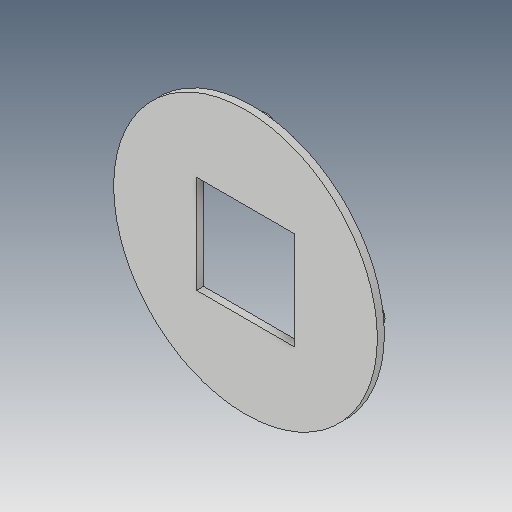
# Autodesk Inventor part: 200_Lambdaplatte_2_conterplate
Saved by Autodesk Inventor 2019 (Build 230136000, 136)
## iProperties
Created: 2019-07-08
Part Number: 200_Lambdaplatte_2_conterplate
Material: Generic
Document SubType Name: Modeling
Designer: diederichbenedict
Density: 1 g/cm^3
Appearance: Default
Author: diederichbenedict
Autodesk Inventor part; units mm, degrees
ref_plane "YZ Plane" through (0, 0, 0) normal (1, 0, 0) x (0, 1, 0)
ref_plane "XZ Plane" through (0, 0, 0) normal (0, 1, 0) x (-1, 0, 0)
ref_plane "XY Plane" through (0, 0, 0) normal (0, 0, 1) x (1, 0, 0)
sketch "Sketch1" plane through (0, 0, 0) normal (0, 0, 1) x (1, 0, 0)
  circle A0 centre (-7.7782, 0) radius 0.9 construction
  circle A1 centre (7.7782, 0) radius 0.9 construction
  circle A2 centre (0, -7.7782) radius 0.9 construction
  circle A3 centre (0, 7.7782) radius 0.9 construction
  arc A4 (0, 10) -> (-2.698, 9.6292) centre (0, 0) ccw construction
  arc A5 (-2.698, 9.6292) -> (-5.1958, 8.5442) centre (0, 0) ccw construction
  arc A6 (-5.1958, 8.5442) -> (-7.3084, 6.8255) centre (0, 0) ccw construction
  arc A7 (-7.3084, 6.8255) -> (-8.8789, 4.6007) centre (0, 0) ccw construction
  arc A8 (-8.8789, 4.6007) -> (-9.7908, 2.0346) centre (0, 0) ccw construction
  arc A9 (-9.7908, 2.0346) -> (-9.9767, -0.6824) centre (0, 0) ccw construction
  arc A10 (-9.9767, -0.6824) -> (-9.4226, -3.3488) centre (0, 0) ccw construction
  arc A11 (-9.4226, -3.3488) -> (-8.1697, -5.7668) centre (0, 0) ccw construction
  arc A12 (-8.1697, -5.7668) -> (-6.3109, -7.7571) centre (0, 0) ccw construction
  arc A13 (-6.3109, -7.7571) -> (-3.984, -9.1721) centre (0, 0) ccw construction
  arc A14 (-3.984, -9.1721) -> (-1.3617, -9.9069) centre (0, 0) ccw construction
  arc A15 (-1.3617, -9.9069) -> (1.3617, -9.9069) centre (0, 0) ccw construction
  arc A16 (1.3617, -9.9069) -> (3.984, -9.1721) centre (0, 0) ccw construction
  arc A17 (3.984, -9.1721) -> (6.3109, -7.7571) centre (0, 0) ccw construction
  arc A18 (6.3109, -7.7571) -> (8.1697, -5.7668) centre (0, 0) ccw construction
  arc A19 (8.1697, -5.7668) -> (9.4226, -3.3488) centre (0, 0) ccw construction
  arc A20 (9.4226, -3.3488) -> (9.9767, -0.6824) centre (0, 0) ccw construction
  arc A21 (9.9767, -0.6824) -> (9.7908, 2.0346) centre (0, 0) ccw construction
  arc A22 (9.7908, 2.0346) -> (8.8789, 4.6007) centre (0, 0) ccw construction
  arc A23 (8.8789, 4.6007) -> (7.3084, 6.8255) centre (0, 0) ccw construction
  arc A24 (7.3084, 6.8255) -> (5.1958, 8.5442) centre (0, 0) ccw construction
  arc A25 (5.1958, 8.5442) -> (2.698, 9.6292) centre (0, 0) ccw construction
  arc A26 (2.698, 9.6292) -> (0, 10) centre (0, 0) ccw construction
  circle A27 centre (0, 0) radius 9.4226
  circle A28 centre (7.7782, 0) radius 0.7
  circle A29 centre (0, -7.7782) radius 0.7
  circle A30 centre (-7.7782, 0) radius 0.7
  circle A31 centre (0, 7.7782) radius 0.7
  line L0 (-3.5, -3.5) -> (3.5, -3.5)
  line L1 (3.5, -3.5) -> (3.5, 3.5)
  line L2 (3.5, 3.5) -> (-3.5, 3.5)
  line L3 (-3.5, 3.5) -> (-3.5, -3.5)
  line L4 (-3.5, -3.5) -> (3.5, 3.5) construction
  line L5 (3.5, -3.5) -> (-3.5, 3.5) construction
  line L6 (4.75, 4.75) -> (4.75, -4.75) projected
  line L7 (4.75, -4.75) -> (-4.75, -4.75) projected
  line L8 (-4.75, -4.75) -> (-4.75, 4.75) projected
  line L9 (-4.75, 4.75) -> (4.75, 4.75) projected
  dimension "d0" = 0.2
  dimension "d1" = 0.2
  dimension "d2" = 0.2
  dimension "d3" = 0.2
  dimension "d4" = 7
  dimension "d5" = 7
  constraints: 12 end point, 5 centre point, 2 midpoint, 2 parallel, 1 coincident, 1 horizontal, 1 perpendicular
  measures "d0" radial gap between concentric circles of A1 A28
  measures "d1" radial gap between concentric circles of A2 A29
  measures "d2" radial gap between concentric circles of A0 A30
  measures "d3" radial gap between concentric circles of A3 A31
  measures "d4" distance of L2.end L1.end
  measures "d5" distance of L1.end L0.end
extrude "Extrusion1" add sketch "Sketch1" along normal blind 0.5 contours A27 | L6 L7 L8 L9
sketch "Sketch2" plane through (0, 0, 0.5) normal (0, 0, 1) x (1, 0, 0)
  line L0 (-3.5, -3.5) -> (-3.5, 3.5) projected
  line L1 (-3.5, 3.5) -> (3.5, 3.5) projected
  line L2 (3.5, 3.5) -> (3.5, -3.5) projected
  line L3 (3.5, -3.5) -> (-3.5, -3.5) projected
  circle A0 centre (0, 7.7782) radius 0.7 projected
  circle A1 centre (-7.7782, 0) radius 0.7 projected
  circle A2 centre (0, -7.7782) radius 0.7 projected
  circle A3 centre (7.7782, 0) radius 0.7 projected
  circle A4 centre (0, 0) radius 9.4226 projected
extrude "Extrusion2" add sketch "Sketch2" against normal blind 1.5 contours A0 | A1 | A2 | A3
body "Solid1"
